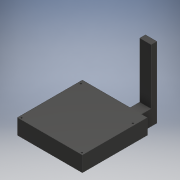
# Autodesk Inventor part: NVIDIA Jetson TX2
Saved by Autodesk Inventor 2017 (Build 210142000, 142)
## iProperties
Created: 2019-06-04
Part Number: NVIDIA Jetson TX2
Material: ABS Plastic
Document SubType Name: Modeling
Designer: Dell
Density: 1.06 g/cm^3
Appearance: Smooth - Black
Author: Dell
Autodesk Inventor part; units mm, degrees
ref_plane "YZ Plane" through (0, 0, 0) normal (1, 0, 0) x (0, 1, 0)
ref_plane "XZ Plane" through (0, 0, 0) normal (0, 1, 0) x (-1, 0, 0)
ref_plane "XY Plane" through (0, 0, 0) normal (0, 0, 1) x (1, 0, 0)
sketch "Sketch1" plane through (0, 0, 0) normal (0, 0, 1) x (1, 0, 0)
  line L0 (0, 0) -> (170, 0)
  line L1 (170, 0) -> (170, 170)
  line L2 (170, 170) -> (0, 170)
  line L3 (0, 170) -> (0, 0)
  circle A0 centre (6, 5) radius 2
  circle A1 centre (164, 5) radius 2
  circle A2 centre (164, 138) radius 2
  circle A3 centre (6, 160) radius 2
  line L4 (6, 5) -> (164, 5) construction
  point P0 (85, 5)
  point P1 (85, 0)
  dimension "d0" = 170
  dimension "d1" = 170
  dimension "d2" = 4
  dimension "d3" = 4
  dimension "d4" = 4
  dimension "d5" = 4
  dimension "d6" = 158
  dimension "d7" = 155
  dimension "d8" = 133
  dimension "d9" = 32
  constraints: 10 end point, 4 centre point, 3 vertical alignment, 2 horizontal, 2 midpoint, 2 parallel, 1 horizontal alignment, 1 perpendicular
  measures "d0" distance of L2.end L1.end
  measures "d1" distance of L1.end L0.end
  measures "d2" diameter of A0
  measures "d3" diameter of A1
  measures "d4" diameter of A2
  measures "d5" diameter of A3
  measures "d6" distance of L4.end L4.start
  measures "d7" distance of L4.start A3.centre
  measures "d8" distance of A2.centre L4.end
  measures "d9" distance from line of A2.centre L2
extrude "Extrusion1" add sketch "Sketch1" along normal blind 40
sketch "Sketch2" plane through (0, 0, 40) normal (0, 0, 1) x (1, 0, 0)
  line L0 (170, 170) -> (0, 170) projected
  line L1 (125, 170) -> (155, 170)
  line L2 (155, 170) -> (155, 210)
  line L3 (155, 210) -> (125, 210)
  line L4 (125, 210) -> (125, 170)
  line L5 (170, 0) -> (170, 170) projected
  point P0 (0, 0)
  dimension "d12" = 30
  dimension "d13" = 40
  dimension "d14" = 15
  constraints: 8 end point, 2 parallel, 1 horizontal, 1 perpendicular, 1 point on line
  measures "d12" distance of L3.end L2.end
  measures "d13" distance of L2.end L1.end
  measures "d14" distance between parallel lines of L5 L2
extrude "Extrusion2" add sketch "Sketch2" against normal blind 40 and the other way blind 145
sketch "Sketch3" plane through (155, 170, 0) normal (1, 0, 0) x (0, 0, -1)
  line L0 (-185, 0) -> (-40, 0) projected
  line L1 (-185, 0) -> (-40, 0)
  line L2 (-40, 0) -> (-40, 25)
  line L3 (-40, 25) -> (-185, 25)
  line L4 (-185, 25) -> (-185, 0)
  point P0 (0, -170)
  dimension "d19" = 25
  constraints: 8 end point, 2 parallel, 1 horizontal, 1 perpendicular, 1 vertical alignment
  measures "d19" distance between parallel lines of L0 L3
extrude "Extrusion3" cut sketch "Sketch3" against normal through all
body "Solid1"
